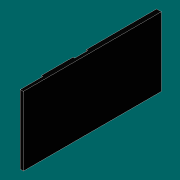
# Autodesk Inventor part: sides
Saved by Autodesk Inventor 2016 SP1 (Build 200210100, 210)
## iProperties
Created: 2015-10-13
Part Number: sides
Material: PC/ABS Plastic
Document SubType Name: Modeling
Designer: Sawaiz
Density: 0.357273 g/cm^3
Appearance: Smooth - Black
Author: Sawaiz
Autodesk Inventor part; units mm, degrees
ref_plane "YZ Plane" through (0, 0, 0) normal (1, 0, 0) x (0, 1, 0)
ref_plane "XZ Plane" through (0, 0, 0) normal (0, 1, 0) x (-1, 0, 0)
ref_plane "XY Plane" through (0, 0, 0) normal (0, 0, 1) x (1, 0, 0)
sketch "Sketch1" plane through (0, 0, 0) normal (0, 1, 0) x (-1, 0, 0)
  line L0 (-136.525, 68.2625) -> (136.525, 68.2625)
  line L1 (136.525, 68.2625) -> (136.525, -68.2625)
  line L2 (136.525, -68.2625) -> (-136.525, -68.2625)
  line L3 (-136.525, -68.2625) -> (-136.525, 68.2625)
  line L4 (-136.525, 68.2625) -> (136.525, -68.2625) construction
  line L5 (136.525, 68.2625) -> (-136.525, -68.2625) construction
  point P0 (0, 0)
  dimension "d0" = 273.05
  dimension "d1" = 136.525
  constraints: 12 end point, 2 midpoint, 2 parallel, 1 horizontal, 1 perpendicular
  measures "d0" distance of L1.end L2.end
  measures "d1" distance of L0.end L1.end
extrude "Extrusion1" add sketch "Sketch1" along normal blind 9.525
sketch "Sketch8" plane through (0, 0, 0) normal (0, -1, 0) x (1, 0, 0)
  line L0 (136.525, 68.2625) -> (-136.525, 68.2625) projected
  line L1 (-136.525, 68.2625) -> (-136.525, -68.2625) projected
  line L2 (-136.525, -68.2625) -> (136.525, -68.2625) projected
  line L3 (136.525, -68.2625) -> (136.525, 68.2625) projected
  line L4 (-136.525, 68.2625) -> (136.525, 68.2625) projected
  line L5 (136.525, 68.2625) -> (91.4073, 68.2625)
  line L6 (91.4073, 68.2625) -> (91.4073, -68.2625)
  line L7 (91.4073, -68.2625) -> (136.525, -68.2625)
  line L8 (136.525, -68.2625) -> (136.525, 68.2625)
  line L9 (136.525, -68.2625) -> (-136.525, -68.2625) projected
  line L10 (2.5072, 68.2625) -> (28.701, 68.2625)
  line L11 (28.701, 68.2625) -> (28.701, -68.2625)
  line L12 (28.701, -68.2625) -> (2.5073, -68.2625)
  line L13 (2.5073, -68.2625) -> (2.5072, 68.2625)
  point P0 (0, 0)
  dimension "d40" = 45.1178
  dimension "d43" = 62.7062
  dimension "d44" = 26.1938
  constraints: 16 end point, 4 parallel, 3 point on line, 2 horizontal, 2 perpendicular
  measures "d40" distance between parallel lines of L3 L6
  measures "d43" distance between parallel lines of L6 L11
  measures "d44" distance between parallel lines of L11 L13
extrude "Extrusion5" cut sketch "Sketch8" against normal blind 3.175 contours L3 L2 L6 L0 | L11 L2 L13 L0
equation "\"d0\" = depth"
equation "\"d1\" = height + 1.5 * internalAcrylicThickness"
equation "\"d2\" = acrylicThickness"
equation "\"d40\" = fresnelThickness + 2 * internalAcrylicThickness + aerogelThickness + centerThickness + moduleSlotClearence"
equation "\"d43\" = -2 * internalAcrylicThickness + focalLength - moduleSlotClearence"
equation "\"d44\" = sensorHolderDepth + internalAcrylicThickness + moduleSlotClearence"
equation "\"d41\" = 0.5 * internalAcrylicThickness"
equation "\"acrylicThickness\" = 9.525"
equation "\"depth\" = 273.05"
equation "\"height\" = 127"
equation "\"fresnelThickness\" = 0.1"
equation "\"focalLength\" = 76.2"
equation "\"centerThickness\" = 1.524"
equation "\"sensorHolderDepth\" = 19.05"
equation "\"internalAcrylicThickness\" = 6.35"
equation "\"frameAcrylicThickness\" = 9.525"
equation "\"width\" = 127"
equation "\"mirrorAngle\" = 5deg"
equation "\"detectorWidth\" = 52"
equation "\"detectorHeight\" = 52"
equation "\"mirrorThickness\" = 3.175"
equation "\"ior\" = 1.49"
equation "\"fresnelAngle\" = 90deg"
equation "\"fresnelEffectiveDiameter\" = 152.4"
equation "\"oRingWidth\" = 1.5875"
equation "\"aerogelClearence\" = 3.175"
equation "\"backplanePCBHeight\" = 76.2"
equation "\"backplaneHoleOffsett\" = 6.35"
equation "\"backplanePCBWidth\" = 76.2"
equation "\"backplanePostionOffsett\" = 12.7"
equation "\"moduleSlotClearence\" = 0.79375"
equation "\"aerogelThickness\" = 30"
body "Solid1"
